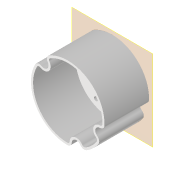
# Autodesk Inventor part: Anglerfish_Batterycase
Saved by Autodesk Inventor 2022 (Build 260153000, 153)
## iProperties
Created: 2022-10-04
Part Number: Anglerfish_Batterycase
Material: Generisch
Document SubType Name: Modeling
Designer: UC2
Density: 1 g/cm^3
Appearance: Vorgabe
Author: UC2
Autodesk Inventor part; units mm, degrees
ref_plane "YZ Plane" through (0, 0, 0) normal (1, 0, 0) x (0, 1, 0)
ref_plane "XZ Plane" through (0, 0, 0) normal (0, 1, 0) x (-1, 0, 0)
ref_plane "XY Plane" through (0, 0, 0) normal (0, 0, 1) x (1, 0, 0)
ref_plane "Arbeitsebene1" through (0, 0, 0) normal (0, 0, 1) x (1, 0, 0)
sketch "Skizze1" plane through (0, 0, 0) normal (0, 0, 1) x (1, 0, 0)
  arc A0 (22.7625, -3.9398) -> (25.9854, -0.8716) centre (22.8122, -0.7652) ccw projected
  arc A1 (25.9854, -0.8716) -> (-13.1449, 22.4324) centre (0, 0) ccw projected
  arc A2 (-13.1449, 22.4324) -> (-14.1536, 17.8908) centre (-11.5397, 19.693) ccw projected
  arc A3 (-18.5446, 13.2855) -> (-14.1536, 17.8908) centre (-16.8293, 16.046) ccw projected
  arc A4 (-18.5446, 13.2855) -> (-23.033, 12.0616) centre (-20.2203, 10.5887) ccw projected
  arc A5 (-23.033, 12.0616) -> (-0.3346, -25.9978) centre (0, 0) ccw projected
  arc A6 (-0.3346, -25.9978) -> (2.8797, -22.9216) centre (-0.2937, -22.8231) ccw projected
  arc A7 (8.8966, -21.32) -> (2.8797, -22.9216) centre (6.1282, -23.0224) ccw projected
  arc A8 (8.8966, -21.32) -> (13.215, -22.3912) centre (11.6012, -19.6569) ccw projected
  arc A9 (13.215, -22.3912) -> (21.7536, -14.2401) centre (0, 0) ccw projected
  arc A10 (21.7536, -14.2401) -> (20.8833, -9.8763) centre (19.0971, -12.5012) ccw projected
  arc A11 (22.7625, -3.9398) -> (20.8833, -9.8763) centre (22.7117, -7.1894) ccw projected
  line L0 (15.6075, -13.9435) -> (-2.8275, -13.9435) projected
  arc A12 (-2.8275, -8.8258) -> (-2.8275, -13.9435) centre (-2.8275, -11.3847) ccw projected
  line L1 (-2.8275, -8.8258) -> (15.6075, -8.8258) projected
  arc A13 (15.6075, -13.9435) -> (15.6075, -8.8258) centre (15.6075, -11.3847) ccw projected
  line L2 (15.5975, 8.4145) -> (-2.8205, 8.4145) projected
  arc A14 (-2.8205, 13.5462) -> (-2.8205, 8.4145) centre (-2.8205, 10.9803) ccw projected
  line L3 (-2.8205, 13.5462) -> (15.5975, 13.5462) projected
  arc A15 (15.5975, 8.4145) -> (15.5975, 13.5462) centre (15.5975, 10.9803) ccw projected
  circle A16 centre (10, -17.5) radius 3.25 projected
  circle A17 centre (-10, 17.5) radius 3.25 projected
  circle A18 centre (10, 17.5) radius 3.25 projected
  circle A19 centre (-10, -17.5) radius 3.25 projected
  circle A20 centre (-10, 17.5) radius 1.4
  circle A21 centre (10, 17.5) radius 1.4
  circle A22 centre (10, -17.5) radius 1.4
  circle A23 centre (-10, -17.5) radius 1.4
  point P0 (0, 0)
  dimension "d0" = 2.8
  dimension "d1" = 2.8
  dimension "d2" = 2.8
  dimension "d3" = 2.8
  constraints: 4 centre point, 4 coincident
  measures "d0" diameter of A20
  measures "d1" diameter of A21
  measures "d2" diameter of A22
  measures "d3" diameter of A23
extrude "Extrusion1" add sketch "Skizze1" along normal blind 1.5 contours A11 A10 A9 A8 A7 A6 A5 A4 A3 A2 A1 A0 | L0 A12 L1 A13 | L2 A14 L3 A15 | A16 | A17 | A18 | A19
sketch "Skizze2" plane through (0, 0, 1.5) normal (0, 0, 1) x (1, 0, 0)
  arc A0 (13.215, -22.3912) -> (21.7536, -14.2401) centre (0, 0) ccw projected
  arc A1 (21.7536, -14.2401) -> (20.8833, -9.8763) centre (19.0971, -12.5012) ccw projected
  arc A2 (22.7625, -3.9398) -> (20.8833, -9.8763) centre (22.7117, -7.1894) ccw projected
  arc A3 (22.7625, -3.9398) -> (25.9854, -0.8716) centre (22.8122, -0.7652) ccw projected
  arc A4 (25.9854, -0.8716) -> (-13.1449, 22.4324) centre (0, 0) ccw projected
  arc A5 (-13.1449, 22.4324) -> (-14.1536, 17.8908) centre (-11.5397, 19.693) ccw projected
  arc A6 (-18.5446, 13.2855) -> (-14.1536, 17.8908) centre (-16.8293, 16.046) ccw projected
  arc A7 (-18.5446, 13.2855) -> (-23.033, 12.0616) centre (-20.2203, 10.5887) ccw projected
  arc A8 (-23.033, 12.0616) -> (-0.3346, -25.9978) centre (0, 0) ccw projected
  arc A9 (-0.3346, -25.9978) -> (2.8797, -22.9216) centre (-0.2937, -22.8231) ccw projected
  arc A10 (8.8966, -21.32) -> (2.8797, -22.9216) centre (6.1282, -23.0224) ccw projected
  arc A11 (8.8966, -21.32) -> (13.215, -22.3912) centre (11.6012, -19.6569) ccw projected
  circle A12 centre (10, -17.5) radius 1.4 projected
  circle A13 centre (-10, 17.5) radius 1.4 projected
  circle A14 centre (10, 17.5) radius 1.4 projected
  circle A15 centre (-10, -17.5) radius 1.4 projected
  arc A16 (24.4862, -0.8213) -> (-12.3865, 21.1382) centre (0, 0) ccw
  arc A17 (22.786, -2.44) -> (24.4862, -0.8213) centre (22.8122, -0.7652) ccw
  arc A18 (22.786, -2.44) -> (20.0395, -11.1164) centre (22.7117, -7.1894) ccw
  arc A19 (20.4986, -13.4186) -> (20.0395, -11.1164) centre (19.0971, -12.5012) ccw
  arc A20 (12.4525, -21.0994) -> (20.4986, -13.4186) centre (0, 0) ccw
  arc A21 (10.1744, -20.5343) -> (12.4525, -21.0994) centre (11.6012, -19.6569) ccw
  arc A22 (10.1744, -20.5343) -> (1.3805, -22.8751) centre (6.1282, -23.0224) ccw
  arc A23 (-0.3153, -24.498) -> (1.3805, -22.8751) centre (-0.2937, -22.8231) ccw
  arc A24 (-21.7041, 11.3658) -> (-0.3153, -24.498) centre (0, 0) ccw
  arc A25 (-19.3362, 12.0114) -> (-21.7041, 11.3658) centre (-20.2203, 10.5887) ccw
  arc A26 (-19.3362, 12.0114) -> (-12.9187, 18.7423) centre (-16.8293, 16.046) ccw
  arc A27 (-12.3865, 21.1382) -> (-12.9187, 18.7423) centre (-11.5397, 19.693) ccw
  point P0 (0, 0)
  dimension "d6" = 1.5
  constraints: 24 point on circle, 12 centre point, 11 other
  measures "d6" radial gap between concentric circles of A4 A16
extrude "Extrusion2" add sketch "Skizze2" along normal blind 30 contours A11 A10 A9 A8 A7 A6 A5 A4 A3 A2 A1 A0
